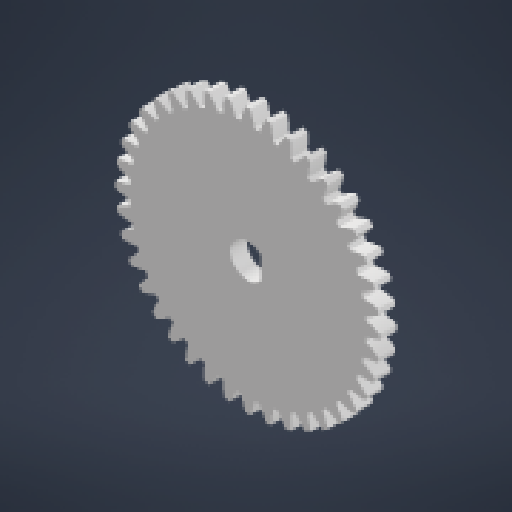
# Autodesk Inventor part: Central_axel_Gear
Saved by Autodesk Inventor 2026 (Build 300175050, 175E)
## iProperties
Created: 2026-04-30
Part Number: Central_axel_Gear
Material: Generic
Document SubType Name: Modeling
Designer: sniel
Density: 1 g/cm^3
Appearance: Default
Author: sniel
Autodesk Inventor part; units mm, degrees
ref_plane "YZ Plane" through (0, 0, 0) normal (1, 0, 0) x (0, 1, 0)
ref_plane "XZ Plane" through (0, 0, 0) normal (0, 1, 0) x (-1, 0, 0)
ref_plane "XY Plane" through (0, 0, 0) normal (0, 0, 1) x (1, 0, 0)
sketch "Sketch1" plane through (0, 0, 0) normal (0, 0, 1) x (1, 0, 0)
  circle A0 centre (0, 0) radius 4.1
  line L0 (0, 0) -> (4.1, 0)
  line L1 (4.1, 0) -> (3.1, 0)
  line L2 (3.1, 0) -> (3.1, -2.6833)
  line L3 (3.1, 0) -> (3.1, 2.6833)
  arc A1 (-10.4029, -26.5793) -> (-10.469, -30.1901) centre (6.3619, -28.6922) ccw
  arc A2 (-10.469, -30.1901) -> (-9.2757, -30.5779) centre (0, 0) ccw
  arc A3 (-9.2757, -30.5779) -> (-7.2068, -27.6178) centre (-22.0117, -19.473) ccw
  arc A4 (-7.2068, -27.6178) -> (-6.1169, -27.8794) centre (0, 0) ccw
  arc A5 (-6.1169, -27.8794) -> (-5.6174, -31.4562) centre (10.772, -27.3437) ccw
  arc A6 (-5.6174, -31.4562) -> (-4.3781, -31.6524) centre (0, 0) ccw
  arc A7 (-4.3781, -31.6524) -> (-2.7977, -28.4052) centre (-18.6944, -22.6767) ccw
  arc A8 (-2.7977, -28.4052) -> (-1.6803, -28.4931) centre (0, 0) ccw
  arc A9 (-1.6803, -28.4931) -> (-0.6274, -31.9476) centre (14.9169, -25.322) ccw
  arc A10 (-0.6274, -31.9476) -> (0.6274, -31.9476) centre (0, 0) ccw
  arc A11 (0.6274, -31.9476) -> (1.6803, -28.4931) centre (-14.9169, -25.322) ccw
  arc A12 (1.6803, -28.4931) -> (2.7977, -28.4052) centre (0, 0) ccw
  arc A13 (2.7977, -28.4052) -> (4.3781, -31.6524) centre (18.6944, -22.6767) ccw
  arc A14 (4.3781, -31.6524) -> (5.6174, -31.4562) centre (0, 0) ccw
  arc A15 (5.6174, -31.4562) -> (6.1169, -27.8794) centre (-10.772, -27.3437) ccw
  arc A16 (6.1169, -27.8794) -> (7.2068, -27.6178) centre (0, 0) ccw
  arc A17 (7.2068, -27.6178) -> (9.2757, -30.5779) centre (22.0117, -19.473) ccw
  arc A18 (9.2757, -30.5779) -> (10.469, -30.1901) centre (0, 0) ccw
  arc A19 (10.469, -30.1901) -> (10.4029, -26.5793) centre (-6.3619, -28.6922) ccw
  arc A20 (10.4029, -26.5793) -> (11.4384, -26.1504) centre (0, 0) ccw
  arc A21 (11.4384, -26.1504) -> (13.9449, -28.7504) centre (24.7869, -15.7899) ccw
  arc A22 (13.9449, -28.7504) -> (15.0629, -28.1807) centre (0, 0) ccw
  arc A23 (15.0629, -28.1807) -> (14.4328, -24.6247) centre (-1.7951, -29.3341) ccw
  arc A24 (14.4328, -24.6247) -> (15.3884, -24.0391) centre (0, 0) ccw
  arc A25 (15.3884, -24.0391) -> (18.2708, -26.2149) centre (26.9519, -11.718) ccw
  arc A26 (18.2708, -26.2149) -> (19.2859, -25.4774) centre (0, 0) ccw
  arc A27 (19.2859, -25.4774) -> (18.1072, -22.0637) centre (2.8159, -29.2538) ccw
  arc A28 (18.1072, -22.0637) -> (18.9595, -21.3358) centre (0, 0) ccw
  arc A29 (18.9595, -21.3358) -> (22.1468, -23.034) centre (28.4531, -7.3575) ccw
  arc A30 (22.1468, -23.034) -> (23.034, -22.1468) centre (0, 0) ccw
  arc A31 (23.034, -22.1468) -> (21.3358, -18.9595) centre (7.3575, -28.4531) ccw
  arc A32 (21.3358, -18.9595) -> (22.0637, -18.1072) centre (0, 0) ccw
  arc A33 (22.0637, -18.1072) -> (25.4774, -19.2859) centre (29.2538, -2.8159) ccw
  arc A34 (25.4774, -19.2859) -> (26.2149, -18.2708) centre (0, 0) ccw
  arc A35 (26.2149, -18.2708) -> (24.0391, -15.3884) centre (11.718, -26.9519) ccw
  arc A36 (24.0391, -15.3884) -> (24.6247, -14.4328) centre (0, 0) ccw
  arc A37 (24.6247, -14.4328) -> (28.1807, -15.0629) centre (29.3341, 1.7951) ccw
  arc A38 (28.1807, -15.0629) -> (28.7504, -13.9449) centre (0, 0) ccw
  arc A39 (28.7504, -13.9449) -> (26.1504, -11.4384) centre (15.7899, -24.7869) ccw
  arc A40 (26.1504, -11.4384) -> (26.5793, -10.4029) centre (0, 0) ccw
  arc A41 (26.5793, -10.4029) -> (30.1901, -10.469) centre (28.6922, 6.3619) ccw
  arc A42 (30.1901, -10.469) -> (30.5779, -9.2757) centre (0, 0) ccw
  arc A43 (30.5779, -9.2757) -> (27.6178, -7.2068) centre (19.473, -22.0117) ccw
  arc A44 (27.6178, -7.2068) -> (27.8794, -6.1169) centre (0, 0) ccw
  arc A45 (27.8794, -6.1169) -> (31.4562, -5.6174) centre (27.3437, 10.772) ccw
  arc A46 (31.4562, -5.6174) -> (31.6524, -4.3781) centre (0, 0) ccw
  arc A47 (31.6524, -4.3781) -> (28.4052, -2.7977) centre (22.6767, -18.6944) ccw
  arc A48 (28.4052, -2.7977) -> (28.4931, -1.6803) centre (0, 0) ccw
  arc A49 (28.4931, -1.6803) -> (31.9476, -0.6274) centre (25.322, 14.9169) ccw
  arc A50 (31.9476, -0.6274) -> (31.9476, 0.6274) centre (0, 0) ccw
  arc A51 (31.9476, 0.6274) -> (28.4931, 1.6803) centre (25.322, -14.9169) ccw
  arc A52 (28.4931, 1.6803) -> (28.4052, 2.7977) centre (0, 0) ccw
  arc A53 (28.4052, 2.7977) -> (31.6524, 4.3781) centre (22.6767, 18.6944) ccw
  arc A54 (31.6524, 4.3781) -> (31.4562, 5.6174) centre (0, 0) ccw
  arc A55 (31.4562, 5.6174) -> (27.8794, 6.1169) centre (27.3437, -10.772) ccw
  arc A56 (27.8794, 6.1169) -> (27.6178, 7.2068) centre (0, 0) ccw
  arc A57 (27.6178, 7.2068) -> (30.5779, 9.2757) centre (19.473, 22.0117) ccw
  arc A58 (30.5779, 9.2757) -> (30.1901, 10.469) centre (0, 0) ccw
  arc A59 (30.1901, 10.469) -> (26.5793, 10.4029) centre (28.6922, -6.3619) ccw
  arc A60 (26.5793, 10.4029) -> (26.1504, 11.4384) centre (0, 0) ccw
  arc A61 (26.1504, 11.4384) -> (28.7504, 13.9449) centre (15.7899, 24.7869) ccw
  arc A62 (28.7504, 13.9449) -> (28.1807, 15.0629) centre (0, 0) ccw
  arc A63 (28.1807, 15.0629) -> (24.6247, 14.4328) centre (29.3341, -1.7951) ccw
  arc A64 (24.6247, 14.4328) -> (24.0391, 15.3884) centre (0, 0) ccw
  arc A65 (24.0391, 15.3884) -> (26.2149, 18.2708) centre (11.718, 26.9519) ccw
  arc A66 (26.2149, 18.2708) -> (25.4774, 19.2859) centre (0, 0) ccw
  arc A67 (25.4774, 19.2859) -> (22.0637, 18.1072) centre (29.2538, 2.8159) ccw
  arc A68 (22.0637, 18.1072) -> (21.3358, 18.9595) centre (0, 0) ccw
  arc A69 (21.3358, 18.9595) -> (23.034, 22.1468) centre (7.3575, 28.4531) ccw
  arc A70 (23.034, 22.1468) -> (22.1468, 23.034) centre (0, 0) ccw
  arc A71 (22.1468, 23.034) -> (18.9595, 21.3358) centre (28.4531, 7.3575) ccw
  arc A72 (18.9595, 21.3358) -> (18.1072, 22.0637) centre (0, 0) ccw
  arc A73 (18.1072, 22.0637) -> (19.2859, 25.4774) centre (2.8159, 29.2538) ccw
  arc A74 (19.2859, 25.4774) -> (18.2708, 26.2149) centre (0, 0) ccw
  arc A75 (18.2708, 26.2149) -> (15.3884, 24.0391) centre (26.9519, 11.718) ccw
  arc A76 (15.3884, 24.0391) -> (14.4328, 24.6247) centre (0, 0) ccw
  arc A77 (14.4328, 24.6247) -> (15.0629, 28.1807) centre (-1.7951, 29.3341) ccw
  arc A78 (15.0629, 28.1807) -> (13.9449, 28.7504) centre (0, 0) ccw
  arc A79 (13.9449, 28.7504) -> (11.4384, 26.1504) centre (24.7869, 15.7899) ccw
  arc A80 (11.4384, 26.1504) -> (10.4029, 26.5793) centre (0, 0) ccw
  arc A81 (10.4029, 26.5793) -> (10.469, 30.1901) centre (-6.3619, 28.6922) ccw
  arc A82 (10.469, 30.1901) -> (9.2757, 30.5779) centre (0, 0) ccw
  arc A83 (9.2757, 30.5779) -> (7.2068, 27.6178) centre (22.0117, 19.473) ccw
  arc A84 (7.2068, 27.6178) -> (6.1169, 27.8794) centre (0, 0) ccw
  arc A85 (6.1169, 27.8794) -> (5.6174, 31.4562) centre (-10.772, 27.3437) ccw
  arc A86 (5.6174, 31.4562) -> (4.3781, 31.6524) centre (0, 0) ccw
  arc A87 (4.3781, 31.6524) -> (2.7977, 28.4052) centre (18.6944, 22.6767) ccw
  arc A88 (2.7977, 28.4052) -> (1.6803, 28.4931) centre (0, 0) ccw
  arc A89 (1.6803, 28.4931) -> (0.6274, 31.9476) centre (-14.9169, 25.322) ccw
  arc A90 (0.6274, 31.9476) -> (-0.6274, 31.9476) centre (0, 0) ccw
  arc A91 (-0.6274, 31.9476) -> (-1.6803, 28.4931) centre (14.9169, 25.322) ccw
  arc A92 (-1.6803, 28.4931) -> (-2.7977, 28.4052) centre (0, 0) ccw
  arc A93 (-2.7977, 28.4052) -> (-4.3781, 31.6524) centre (-18.6944, 22.6767) ccw
  arc A94 (-4.3781, 31.6524) -> (-5.6174, 31.4562) centre (0, 0) ccw
  arc A95 (-5.6174, 31.4562) -> (-6.1169, 27.8794) centre (10.772, 27.3437) ccw
  arc A96 (-6.1169, 27.8794) -> (-7.2068, 27.6178) centre (0, 0) ccw
  arc A97 (-7.2068, 27.6178) -> (-9.2757, 30.5779) centre (-22.0117, 19.473) ccw
  arc A98 (-9.2757, 30.5779) -> (-10.469, 30.1901) centre (0, 0) ccw
  arc A99 (-10.469, 30.1901) -> (-10.4029, 26.5793) centre (6.3619, 28.6922) ccw
  arc A100 (-10.4029, 26.5793) -> (-11.4384, 26.1504) centre (0, 0) ccw
  arc A101 (-11.4384, 26.1504) -> (-13.9449, 28.7504) centre (-24.7869, 15.7899) ccw
  arc A102 (-13.9449, 28.7504) -> (-15.0629, 28.1807) centre (0, 0) ccw
  arc A103 (-15.0629, 28.1807) -> (-14.4328, 24.6247) centre (1.7951, 29.3341) ccw
  arc A104 (-14.4328, 24.6247) -> (-15.3884, 24.0391) centre (0, 0) ccw
  arc A105 (-15.3884, 24.0391) -> (-18.2708, 26.2149) centre (-26.9519, 11.718) ccw
  arc A106 (-18.2708, 26.2149) -> (-19.2859, 25.4774) centre (0, 0) ccw
  arc A107 (-19.2859, 25.4774) -> (-18.1072, 22.0637) centre (-2.8159, 29.2538) ccw
  arc A108 (-18.1072, 22.0637) -> (-18.9595, 21.3358) centre (0, 0) ccw
  arc A109 (-18.9595, 21.3358) -> (-22.1468, 23.034) centre (-28.4531, 7.3575) ccw
  arc A110 (-22.1468, 23.034) -> (-23.034, 22.1468) centre (0, 0) ccw
  arc A111 (-23.034, 22.1468) -> (-21.3358, 18.9595) centre (-7.3575, 28.4531) ccw
  arc A112 (-21.3358, 18.9595) -> (-22.0637, 18.1072) centre (0, 0) ccw
  arc A113 (-22.0637, 18.1072) -> (-25.4774, 19.2859) centre (-29.2538, 2.8159) ccw
  arc A114 (-25.4774, 19.2859) -> (-26.2149, 18.2708) centre (0, 0) ccw
  arc A115 (-26.2149, 18.2708) -> (-24.0391, 15.3884) centre (-11.718, 26.9519) ccw
  arc A116 (-24.0391, 15.3884) -> (-24.6247, 14.4328) centre (0, 0) ccw
  arc A117 (-24.6247, 14.4328) -> (-28.1807, 15.0629) centre (-29.3341, -1.7951) ccw
  arc A118 (-28.1807, 15.0629) -> (-28.7504, 13.9449) centre (0, 0) ccw
  arc A119 (-28.7504, 13.9449) -> (-26.1504, 11.4384) centre (-15.7899, 24.7869) ccw
  arc A120 (-26.1504, 11.4384) -> (-26.5793, 10.4029) centre (0, 0) ccw
  arc A121 (-26.5793, 10.4029) -> (-30.1901, 10.469) centre (-28.6922, -6.3619) ccw
  arc A122 (-30.1901, 10.469) -> (-30.5779, 9.2757) centre (0, 0) ccw
  arc A123 (-30.5779, 9.2757) -> (-27.6178, 7.2068) centre (-19.473, 22.0117) ccw
  arc A124 (-27.6178, 7.2068) -> (-27.8794, 6.1169) centre (0, 0) ccw
  arc A125 (-27.8794, 6.1169) -> (-31.4562, 5.6174) centre (-27.3437, -10.772) ccw
  arc A126 (-31.4562, 5.6174) -> (-31.6524, 4.3781) centre (0, 0) ccw
  arc A127 (-31.6524, 4.3781) -> (-28.4052, 2.7977) centre (-22.6767, 18.6944) ccw
  arc A128 (-28.4052, 2.7977) -> (-28.4931, 1.6803) centre (0, 0) ccw
  arc A129 (-28.4931, 1.6803) -> (-31.9476, 0.6274) centre (-25.322, -14.9169) ccw
  arc A130 (-31.9476, 0.6274) -> (-31.9476, -0.6274) centre (0, 0) ccw
  arc A131 (-31.9476, -0.6274) -> (-28.4931, -1.6803) centre (-25.322, 14.9169) ccw
  arc A132 (-28.4931, -1.6803) -> (-28.4052, -2.7977) centre (0, 0) ccw
  arc A133 (-28.4052, -2.7977) -> (-31.6524, -4.3781) centre (-22.6767, -18.6944) ccw
  arc A134 (-31.6524, -4.3781) -> (-31.4562, -5.6174) centre (0, 0) ccw
  arc A135 (-31.4562, -5.6174) -> (-27.8794, -6.1169) centre (-27.3437, 10.772) ccw
  arc A136 (-27.8794, -6.1169) -> (-27.6178, -7.2068) centre (0, 0) ccw
  arc A137 (-27.6178, -7.2068) -> (-30.5779, -9.2757) centre (-19.473, -22.0117) ccw
  arc A138 (-30.5779, -9.2757) -> (-30.1901, -10.469) centre (0, 0) ccw
  arc A139 (-30.1901, -10.469) -> (-26.5793, -10.4029) centre (-28.6922, 6.3619) ccw
  arc A140 (-26.5793, -10.4029) -> (-26.1504, -11.4384) centre (0, 0) ccw
  arc A141 (-26.1504, -11.4384) -> (-28.7504, -13.9449) centre (-15.7899, -24.7869) ccw
  arc A142 (-28.7504, -13.9449) -> (-28.1807, -15.0629) centre (0, 0) ccw
  arc A143 (-28.1807, -15.0629) -> (-24.6247, -14.4328) centre (-29.3341, 1.7951) ccw
  arc A144 (-24.6247, -14.4328) -> (-24.0391, -15.3884) centre (0, 0) ccw
  arc A145 (-24.0391, -15.3884) -> (-26.2149, -18.2708) centre (-11.718, -26.9519) ccw
  arc A146 (-26.2149, -18.2708) -> (-25.4774, -19.2859) centre (0, 0) ccw
  arc A147 (-25.4774, -19.2859) -> (-22.0637, -18.1072) centre (-29.2538, -2.8159) ccw
  arc A148 (-22.0637, -18.1072) -> (-21.3358, -18.9595) centre (0, 0) ccw
  arc A149 (-21.3358, -18.9595) -> (-23.034, -22.1468) centre (-7.3575, -28.4531) ccw
  arc A150 (-23.034, -22.1468) -> (-22.1468, -23.034) centre (0, 0) ccw
  arc A151 (-22.1468, -23.034) -> (-18.9595, -21.3358) centre (-28.4531, -7.3575) ccw
  arc A152 (-18.9595, -21.3358) -> (-18.1072, -22.0637) centre (0, 0) ccw
  arc A153 (-18.1072, -22.0637) -> (-19.2859, -25.4774) centre (-2.8159, -29.2538) ccw
  arc A154 (-19.2859, -25.4774) -> (-18.2708, -26.2149) centre (0, 0) ccw
  arc A155 (-18.2708, -26.2149) -> (-15.3884, -24.0391) centre (-26.9519, -11.718) ccw
  arc A156 (-15.3884, -24.0391) -> (-14.4328, -24.6247) centre (0, 0) ccw
  arc A157 (-14.4328, -24.6247) -> (-15.0629, -28.1807) centre (1.7951, -29.3341) ccw
  arc A158 (-15.0629, -28.1807) -> (-13.9449, -28.7504) centre (0, 0) ccw
  arc A159 (-13.9449, -28.7504) -> (-11.4384, -26.1504) centre (-24.7869, -15.7899) ccw
  arc A160 (-11.4384, -26.1504) -> (-10.4029, -26.5793) centre (0, 0) ccw
  point P0 (0, 0)
  point P1 (2.1, -3.5214)
  point P2 (2.1, 3.5214)
  dimension "d2" = 8.2
  dimension "d4" = 1
  constraints: 325 point on circle, 161 centre point, 8 end point, 2 point on line, 1 horizontal, 1 perpendicular
  measures "d2" diameter of A0
  measures "d4" distance of L0.end L1.end
extrude "Extrusion1" add sketch "Sketch1" along normal blind 4 contours L0 L3 A0 | A0 L2 L0 | A160 A159 A158 A157 A156 A155 A154 A153 A152 A151 A150 A149 A148 A147 A146 A145 A144 A143 A142 A141 A140 A139 A138 A137 A136 A135 A134 A133 A132 A131 A130 A129 A128 A127 A126 A125 A124 A123 A122 A121 A120 A119 A118 A117 A116 A115 A114 A113 A112 A111 A110 A109 A108 A107 A106 A105 A104 A103 A102 A101 A100 A99 A98 A97 A96 A95 A94 A93 A92 A91 A90 A89 A88 A87 A86 A85 A84 A83 A82 A81 A80 A79 A78 A77 A76 A75 A74 A73 A72 A71 A70 A69 A68 A67 A66 A65 A64 A63 A62 A61 A60 A59 A58 A57 A56 A55 A54 A53 A52 A51 A50 A49 A48 A47 A46 A45 A44 A43 A42 A41 A40 A39 A38 A37 A36 A35 A34 A33 A32 A31 A30 A29 A28 A27 A26 A25 A24 A23 A22 A21 A20 A19 A18 A17 A16 A15 A14 A13 A12 A11 A10 A9 A8 A7 A6 A5 A4 A3 A2 A1
body "Solid1"
